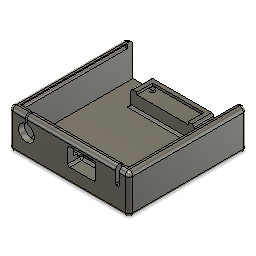
SyncLedStripHousing (Autodesk Fusion 360 design; units mm, degrees)
Autodesk Fusion 360 part; units mm, degrees
sketch "lipo battery" plane through (0, 0, 0) normal (0, 1, 0) x (1, 0, 0)
  line L0 (0, 0) -> (51, 0)
  line L1 (51, 0) -> (51, 34)
  line L2 (51, 34) -> (0, 34)
  line L3 (0, 34) -> (0, 0)
  dimension "d1" = 51
  dimension "d2" = 34
  constraint horizontal L0
  constraint vertical L1
  constraint horizontal L2
  constraint vertical L3
  constraint coincident L0.start L3.end
  measures "d1" distance of L0.start L0.end
  measures "d2" distance of L0.start L2.end
  measures "d159" distance of L0.start
extrude "Extrude1" add sketch "lipo battery" along normal blind 5.5 makes body 1
sketch "Lolin board" plane through (0, 0, 0) normal (0, 1, 0) x (1, 0, 0)
  line L0 (10, -5) -> (36, -5)
  line L1 (36, -5) -> (36, 45)
  line L2 (36, 45) -> (10, 45)
  line L3 (10, 45) -> (10, -5)
  line L4 (33.0596, -5) -> (25.0596, -5)
  line L5 (25.0596, -5) -> (25.0596, 1)
  line L6 (25.0596, 1) -> (33.0596, 1)
  line L7 (33.0596, 1) -> (33.0596, -5)
  line L8 (10, -5) -> (19.5, -5)
  line L9 (19.5, -5) -> (19.5, 3)
  line L10 (19.5, 3) -> (10, 3)
  line L11 (10, 3) -> (10, -5)
  circle A0 centre (12.4, 42.6) radius 1
  circle A1 centre (33.6, 3.5) radius 1
  dimension "d5" = 26
  dimension "d6" = 50
  dimension "d7" = 8
  dimension "d8" = 6
  dimension "d9" = 9.5
  dimension "d10" = 8
  dimension "d11" = 2
  dimension "d12" = 2
  constraint horizontal L0
  constraint vertical L1
  constraint horizontal L2
  constraint vertical L3
  constraint horizontal L4
  constraint vertical L5
  constraint horizontal L6
  constraint vertical L7
  constraint coincident L0 L4.start
  constraint horizontal L8
  constraint vertical L9
  constraint horizontal L10
  constraint vertical L11
  measures "d5" distance of L0.start L0.end
  measures "d6" distance of L0.start L2.end
  measures "d7" distance of L4.start L4.end
  measures "d8" distance of L4.start L6.end
  measures "d9" distance of L0.start L8.end
  measures "d10" distance of L0.start L10.end
  measures "d11" diameter of A0
  measures "d12" diameter of A1
extrude "Extrude2" add sketch "Lolin board" against normal blind 1.2 separate body makes body 2
extrude "Extrude3" add sketch "Lolin board" along normal blind 5.7 separate body contours L0 L3 L8 L9 L10 L11 makes body 3
extrude "Extrude4" add sketch "Lolin board" along normal blind 2.3 separate body contours L0 L4 L5 L6 L7 makes body 4
combine "Combine1" operation add target body 2 tool bodies 3 4
move_body "Move1" bodies 2 to x (1, 0, 0) y (0, 1, 0) z (0, 0, 1) at (0, 8, -3)
move_body "Move15" bodies 2 to x (1, 0, 0) y (0, 1, 0) z (0, 0, 1) at (3, 0, 6)
sketch "Housing" plane through (0, 0, 0) normal (0, 1, 0) x (1, 0, 0) in component "Housing"
  line L0 (-2, -10) -> (53, -10)
  line L1 (53, -10) -> (53, 44)
  line L2 (53, 44) -> (-2, 44)
  line L3 (-2, 44) -> (-2, -10)
  line L4 (10, 34) -> (42, 34)
  line L5 (42, 34) -> (42, 44)
  line L6 (42, 44) -> (10, 44)
  line L7 (10, 44) -> (10, 34)
  line L8 (10, -10) -> (42, -10)
  line L9 (42, -10) -> (42, -1)
  line L10 (42, -1) -> (10, -1)
  line L11 (10, -1) -> (10, -10)
  line L12 (-5, -13) -> (56, -13)
  line L13 (56, -13) -> (56, 47)
  line L14 (56, 47) -> (-5, 47)
  line L15 (-5, 47) -> (-5, -13)
  line L16 (39, -10) -> (25, -10)
  line L17 (25, -10) -> (25, -13)
  line L18 (25, -13) -> (39, -13)
  line L19 (39, -13) -> (39, -10)
  dimension "d121" = 3
  dimension "d122" = 14
  constraint horizontal L0
  constraint vertical L1
  constraint horizontal L2
  constraint vertical L3
  constraint horizontal L4
  constraint vertical L5
  constraint horizontal L6
  constraint vertical L7
  constraint coincident L2 L5.end
  constraint horizontal L8
  constraint vertical L9
  constraint horizontal L10
  constraint vertical L11
  constraint coincident L0 L8.start
  constraint horizontal L16
  constraint vertical L17
  constraint horizontal L18
  constraint vertical L19
  constraint coincident L0 L16.start
  measures "d122" distance of L16.start L16.end
extrude "Extrude1'" add sketch "Housing" against normal blind 3 separate body makes body 5 in component "Housing"
extrude "Extrude2'" add sketch "Housing" along normal blind 17 contours L0 L1 L2 L3 L6 L8 L12 L13 L14 L15 L17 L19 | L0 L8 L12 L16 L17 L18 L19 bodies 5 in component "Housing"
extrude "Extrude3'" add sketch "Housing" along normal blind 8 contours L0 L8 L9 L10 L11 L16 | L2 L4 L5 L6 L7 bodies 5 in component "Housing"
combine "Combine1'" operation cut target body 5 tool bodies 2 keep tools in component "Housing"
extrude "Extrude4'" add sketch "Housing" along normal blind 9 separate body contours L0 L8 L12 L16 L17 L18 L19 makes body 6 in component "Housing"
move_face "OffsetFaces1" offset 4 1 faces at (29.6667, 6, 10) on bodies 6 in component "Housing"
move_body "Move1'" bodies 6 to x (1, 0, 0) y (0, 1, 0) z (0, 0, 1) at (0, 5, 0) in component "Housing"
combine "Combine2" operation cut target body 5 tool bodies 6 in component "Housing"
sketch "Lid" plane through (0, 17, 0) normal (0, 1, 0) x (-1, 0, 0) in component "Lid"
  line L0 (-53, 10) -> (2, 10)
  line L1 (2, 10) -> (2, -44)
  line L2 (2, -44) -> (-53, -44)
  line L3 (-53, -44) -> (-53, 10)
  line L4 (5, 13) -> (-56, 13)
  line L5 (-56, 13) -> (-56, -47)
  line L6 (-56, -47) -> (5, -47)
  line L7 (5, -47) -> (5, 13)
  line L8 (5, -47) -> (-56, -47)
  line L9 (-56, -47) -> (-56, 13)
  line L10 (-56, 13) -> (5, 13)
  line L11 (5, 13) -> (5, -47)
  line L12 (2, -44) -> (-53, -44)
  line L13 (-53, -44) -> (-53, 10)
  line L14 (-53, 10) -> (2, 10)
  line L15 (2, 10) -> (2, -44)
  line L16 (-53, -44) -> (-53, -47)
  line L17 (2, -44) -> (2, -47)
  line L18 (-10, -44) -> (-42, -44)
  line L19 (-42, -44) -> (-42, -38)
  line L20 (-42, -38) -> (-10, -38)
  line L21 (-10, -38) -> (-10, -44)
  dimension "d132" = 3
  constraint horizontal L8
  constraint vertical L9
  constraint horizontal L10
  constraint vertical L11
  constraint coincident L4.end L5.start
  constraint coincident L6.end L7.start
  constraint coincident L2.end L3.start
  constraint coincident L6 L16.end
  constraint perpendicular L6 L16
  constraint coincident L1.end L2.start
  constraint coincident L6 L17.end
  constraint perpendicular L6 L17
  constraint horizontal L18
  constraint vertical L19
  constraint horizontal L20
  constraint vertical L21
  constraint coincident L2 L18.start
extrude "Extrude1''" add sketch "Lid" against normal blind 3 separate body contours L0 L1 L2 L3 L12 L13 L14 L15 L19 L20 L21 | L2 L12 L18 L19 L20 L21 makes body 7 in component "Lid"
extrude "Extrude2''" add sketch "Lid" against normal blind 17 contours L2 L6 L8 L12 L16 L17 L18 bodies 7 in component "Lid"
sketch "Sketch2" plane through (0, 0, 10) normal (0, 0, 1) x (1, 0, 0) in component "Lid"
  line L0 (53, 17) -> (-2, 17)
  line L1 (-2, 17) -> (-2, 14)
  line L2 (-2, 14) -> (53, 14)
  line L3 (53, 14) -> (53, 17)
  circle A0 centre (-2, 15.5) radius 1
  circle A1 centre (53, 15.5) radius 1
  dimension "d137" = 2
  dimension "d138" = 2
  constraint midpoint L1 A0.centre
  constraint midpoint L3 A1.centre
  measures "d137" diameter of A0
  measures "d138" diameter of A1
extrude "Extrude3''" add sketch "Sketch2" against normal blind 54 contours L3 A1 | L3 A1 | L1 A0 | L1 A0 bodies 7 in component "Lid"
combine "Combine3" operation cut target body 5 tool bodies 7 keep tools in component "Housing"
move_face "OffsetFaces1'" offset -0.5 1 faces at (-2, 10.3333, -46) on bodies 7 in component "Lid"
move_face "MoveFace1" to x (1, 0, 0) y (0, 1, 0) z (0, 0, 1) at (0.5, 0, 0) 1 faces at (-2.9749, 15.2775, -8) on bodies 7 in component "Lid"
move_face "OffsetFaces2" offset -0.5 1 faces at (53, 10.3333, -46) on bodies 7 in component "Lid"
move_face "MoveFace2" to x (1, 0, 0) y (0, 1, 0) z (0, 0, 1) at (-0.5, 0, 0) 1 faces at (53.4562, 14.6101, -26) on bodies 7 in component "Lid"
move_face "OffsetFaces3" offset -0.5 1 faces at (34.5, 15.1667, 10) on bodies 7 in component "Lid"
fillet "Fillet1" radius 2 4 edges at (-5, 7, -47) (-5, 7, 13) (56, 7, 13) (56, 7, -47) on bodies 5 in component "Housing"
fillet "Fillet2" radius 2 8 edges at (55.4142, -3, 12.4142) (25.5, -3, 13) (-4.4142, -3, 12.4142) (-5, -3, -17) (-4.4142, -3, -46.4142) (25.5, -3, -47) (55.4142, -3, -46.4142) (56, -3, -17) on bodies 5 in component "Housing"
fillet "Fillet1'" radius 1 4 edges at (53.5, 15.5, -44) (-2.5, 15.5, -44) (-2.5, 15.5, 9.5) (53.5, 15.5, 9.5) on bodies 7 in component "Lid"
fillet "Fillet3" radius 1 4 edges at (39, 5, 9.5) (39, 14, 11.5) (25, 14, 11.5) (25, 5, 9.5) on bodies 5 in component "Housing"
fillet "Fillet4" radius 1 4 edges at (42, 8, -39) (42, 8, 5.5) (10, 8, 5.5) (10, 8, -39) on bodies 5 in component "Housing"
fillet "Fillet5" radius 1 6 edges at (42, 0, -39) (26, 0, -34) (42, 0, 5.5) (26, 0, 1) (10, 0, 5.5) (10, 0, -39) on bodies 5 in component "Housing"
fillet "Fillet6" radius 1 5 edges at (39, 6.4, 6) (38.7071, 5.2929, 6) (32, 5, 6) (25.2929, 5.2929, 6) (25, 6.4, 6) on bodies 5 in component "Housing"
extrude "Extrude4''" add sketch "Lid" against normal blind 8.5 contours L2 L12 L18 L19 L20 L21 bodies 7 in component "Lid"
draft "Draft1" angle 5 neutral plane through (42, 17, -44) pull (0, 0, 1) 1 faces at (31.3333, 8.5, -42) on bodies 7 in component "Lid"
fillet "Fillet2'" radius 1 5 edges at (10, 8.7625, -41) (26, 9.0249, -38) (42, 8.7625, -41) (42, 11.5125, -38) (10, 11.5125, -38) on bodies 7 in component "Lid"
fillet "Fillet3'" radius 1 7 edges at (10, 14, -41.5) (10.2929, 14, -38.2929) (26, 14, -38) (41.7071, 14, -38.2929) (42, 14, -41.5) (47.25, 14, -44) (4.25, 14, -44) on bodies 7 in component "Lid"
fillet "Fillet4'" radius 2 1 edges at (25.5, 17, -47) on bodies 7 in component "Lid"
fillet "Fillet7" radius 2 9 edges at (-2.5, 17, -47) (-4.4142, 17, -46.4142) (-5, 17, -17) (-4.4142, 17, 12.4142) (25.5, 17, 13) (55.4142, 17, 12.4142) (56, 17, -17) (55.4142, 17, -46.4142) (53.5, 17, -47) on bodies 5 in component "Housing"
sketch "Sketch1" plane through (0, 17, 0) normal (0, 1, 0) x (-1, 0, 0) in component "Holder"
  line L0 (-52.5, -45) -> (1.5, -45)
  line L1 (1.5, -45) -> (1.5, 9.5)
  line L2 (1.5, 9.5) -> (-52.5, 9.5)
  line L3 (-52.5, 9.5) -> (-52.5, -45)
  line L4 (-56, -15) -> (5, -15)
  line L5 (5, -15) -> (5, 11.0228)
  line L6 (3, 13.0228) -> (-54, 13.0228)
  line L7 (-56, 11.0228) -> (-56, -15)
  arc A0 (5, 11.0228) -> (3, 13.0228) centre (3, 11.0228) ccw
  arc A1 (-54, 13.0228) -> (-56, 11.0228) centre (-54, 11.0228) ccw
  line L8 (7, -15) -> (7, 11.0228)
  arc A2 (7, 11.0228) -> (3, 15.0228) centre (3, 11.0228) ccw
  line L9 (3, 15.0228) -> (-54, 15.0228)
  arc A3 (-54, 15.0228) -> (-58, 11.0228) centre (-54, 11.0228) ccw
  line L10 (-58, 11.0228) -> (-58, -15)
  line L11 (7, -15) -> (-58, -15)
  circle A4 centre (-10, -5) radius 1.5
  circle A5 centre (-41, -5) radius 1.5
  line L12 (3, -15) -> (3, 9.0228)
  line L13 (1, 11.0228) -> (-52, 11.0228)
  line L14 (-54, 9.0228) -> (-54, -15)
  arc A6 (3, 9.0228) -> (1, 11.0228) centre (1, 9.0228) ccw
  arc A7 (-52, 11.0228) -> (-54, 9.0228) centre (-52, 9.0228) ccw
  dimension "d159" = 61
  dimension "d160" = 2
  dimension "d161" = 2
  dimension "d162" = 2
  dimension "d163" = 3
  dimension "d164" = 3
  dimension "d172" = 2
  dimension "d173" = 2
  constraint horizontal L4
  constraint vertical L5
  constraint horizontal L6
  constraint vertical L7
  constraint tangent L5 A0
  constraint tangent L6 A0
  constraint tangent L6 A1
  constraint tangent L7 A1
  constraint perpendicular L10 L11
  constraint parallel L5 L12
  constraint parallel L6 L13
  constraint parallel L7 L14
  constraint tangent L12 A6
  constraint tangent L13 A6
  constraint tangent L13 A7
  constraint tangent L14 A7
  measures "d159" distance of L4.start L4.end
  measures "d160" radius of A0
  measures "d161" radius of A1
  measures "d163" diameter of A4
  measures "d164" diameter of A5
  measures "d172" radius of A6
  measures "d173" radius of A7
extrude "Extrude3'''" add sketch "Sketch1" along normal blind 2 separate body contours L4 L5 L6 L7 A0 A1 L11 L12 L13 L14 A6 A7 | L5 L6 L7 A0 A1 L8 A2 L9 A3 L10 L11 makes body 8 in component "Holder"
extrude "Extrude2'''" add sketch "Sketch1" against normal blind 20 separate body contours L5 L6 L7 A0 A1 L8 A2 L9 A3 L10 L11 makes body 9 in component "Holder"
extrude "Extrude1'''" add sketch "Sketch1" along normal blind 3 separate body contours L1 L2 L3 L4 L11 L12 L13 L14 A6 A7 | L1 L2 L3 L4 L11 | L4 L5 L6 L7 A0 A1 L11 L12 L13 L14 A6 A7 | L5 L6 L7 A0 A1 L8 A2 L9 A3 L10 L11 makes body 10 in component "Holder"
move_body "Move1''" bodies 8 to x (1, 0, 0) y (0, 1, 0) z (0, 0, 1) at (0, -22, 0) in component "Holder"
combine "Combine1''" operation add target body 8 tool bodies 9 10 in component "Holder"
combine "Combine2'" operation cut target body 8 tool bodies 5 7 keep tools in component "Holder"
move_face "OffsetFaces1''" offset -0.5 3 faces at (56, 3.6667, 2.3485) (-5, 3.6667, -6.3257) (16, 10.3333, 13.0228) on bodies 8 in component "Holder"
move_face "OffsetFaces2'" offset -0.5 1 faces at (16.6667, -3, 12.6894) on bodies 8 in component "Holder"
fillet "Fillet1''" radius 2 5 edges at (-7, -5, -1.9886) (-5.8284, -5, 13.8512) (25.5, -5, 15.0228) (56.8284, -5, 13.8512) (58, -5, -1.9886) on bodies 8 in component "Holder"
fillet "Fillet2''" radius 2 5 edges at (-7, 20, -1.9886) (-5.8284, 20, 13.8512) (25.5, 20, 15.0228) (56.8284, 20, 13.8512) (58, 20, -1.9886) on bodies 8 in component "Holder"
fillet "Fillet3''" radius 2 5 edges at (-5.5, -3.5, -1.7386) (-4.9142, -3.5, 12.937) (25.5, -3.5, 13.5228) (55.9142, -3.5, 12.937) (56.5, -3.5, -1.7386) on bodies 8 in component "Holder"
fillet "Fillet4''" radius 2 5 edges at (-5.5, 17, -1.7386) (-4.9142, 17, 12.937) (25.5, 17, 13.5228) (55.9142, 17, 12.937) (56.5, 17, -1.7386) on bodies 8 in component "Holder"
fillet "Fillet5'" radius 1 5 edges at (-3, -5, -2.9886) (-2.4142, -5, 10.437) (25.5, -5, 11.0228) (53.4142, -5, 10.437) (54, -5, -2.9886) on bodies 8 in component "Holder"
chamfer "Chamfer1" distance 2 angle 45 1 edges at (11.3985, 17, -4.4576) on bodies 8 in component "Holder"
chamfer "Chamfer2" distance 2 angle 45 1 edges at (42.3985, 17, -4.4576) on bodies 8 in component "Holder"
fillet "Fillet7'" radius 1 13 edges at (54, -3.75, -15) (54.2929, -4.7071, -15) (55.5, -5, -15) (57.4142, -4.4142, -15) (58, 7.5, -15) (57.4142, 19.4142, -15) (25.5, 20, -15) (-6.4142, 19.4142, -15) (-7, 7.5, -15) (-6.4142, -4.4142, -15) (-4.5, -5, -15) (-3.2929, -4.7071, -15) (-3, -3.75, -15) on bodies 8 in component "Holder"
fillet "Fillet8" radius 0.6 16 edges at (56.5, 6.75, -15) (56.0811, -2.7247, -15) (54.7462, -3.4846, -14.967) (54.134, -3.5, -14.5) (54, -3.5, -2.4886) (53.4142, -3.5, 10.437) (25.5, -3.5, 11.0228) (-2.4142, -3.5, 10.437) (-3, -3.5, -2.4886) (-3.134, -3.5, -14.5) (-3.7462, -3.4846, -14.967) (-5.0811, -2.7247, -15) (-5.5, 6.75, -15) (-4.9142, 16.4142, -15) (25.5, 17, -15) (55.9142, 16.4142, -15) on bodies 8 in component "Holder"
sketch "Buttonhole" plane through (0, 0, 10) normal (0, 0, -1) x (-1, 0, 0)
  arc A0 (-43, 0) -> (-42, 1) centre (-43, 1) ccw
  line L0 (-42, 1) -> (-42, 7)
  arc A1 (-41, 8) -> (-42, 7) centre (-41, 7) ccw
  line L1 (-41, 8) -> (-39, 8)
  line L2 (-39, 8) -> (-39, 13)
  arc A2 (-38, 14) -> (-39, 13) centre (-38, 13) ccw
  line L3 (-38, 14) -> (-26, 14)
  arc A3 (-25, 13) -> (-26, 14) centre (-26, 13) ccw
  line L4 (-25, 13) -> (-25, 8)
  line L5 (-25, 8) -> (-11, 8)
  arc A4 (-10, 7) -> (-11, 8) centre (-11, 7) ccw
  line L6 (-10, 7) -> (-10, 1)
  arc A5 (-10, 1) -> (-9, 0) centre (-9, 1) ccw
  line L7 (-9, 0) -> (2, 0)
  line L8 (2, 0) -> (2, 14.5)
  arc A6 (2, 14.5) -> (2, 16.5) centre (2, 15.5) ccw
  line L9 (2, 17) -> (-53, 17)
  line L10 (-53, 17) -> (-53, 16.5)
  arc A7 (-53, 16.5) -> (-53, 14.5) centre (-53, 15.5) ccw
  line L11 (-53, 14.5) -> (-53, 0)
  line L12 (-53, 0) -> (-43, 0)
  line L13 (1.0045, 14.0126) -> (-8.9955, 14.0126)
  line L14 (-8.9955, 14.0126) -> (-8.9955, 4.0126)
  line L15 (-8.9955, 4.0126) -> (1.0045, 4.0126)
  line L16 (1.0045, 4.0126) -> (1.0045, 14.0126)
  circle A8 centre (-3.9955, 9.0126) radius 4
  line L17 (2, 16.5) -> (2, 17)
  line L18 (-51.0774, 17) -> (-49.0774, 17)
  line L19 (-49.0774, 17) -> (-49.0774, 9.5)
  line L20 (-49.5774, 9) -> (-50.5774, 9)
  line L21 (-51.0774, 9.5) -> (-51.0774, 17)
  arc A9 (-51.0774, 9.5) -> (-50.5774, 9) centre (-50.5774, 9.5) ccw
  arc A10 (-49.5774, 9) -> (-49.0774, 9.5) centre (-49.5774, 9.5) ccw
  line L22 (-4.4955, 12.506) -> (-3.4955, 12.506)
  line L23 (-3.4955, 12.506) -> (-3.4955, 17.506)
  line L24 (-3.4955, 17.506) -> (-4.4955, 17.506)
  line L25 (-4.4955, 17.506) -> (-4.4955, 12.506)
  line L26 (-4.4955, 12.506) -> (-3.4955, 17.506) construction
  line L27 (-3.4955, 12.506) -> (-4.4955, 17.506) construction
  point P0 (-51.0774, 9)
  point P1 (-3.9955, 15.006)
  dimension "d204" = 10
  dimension "d205" = 10
  dimension "d206" = 8
  dimension "d209" = 2
  dimension "d210" = 8
  dimension "d211" = 0.5
  dimension "d212" = 0.5
  dimension "d215" = 1
  dimension "d216" = 5
  constraint horizontal L13
  constraint vertical L14
  constraint horizontal L15
  constraint vertical L16
  constraint horizontal L18
  constraint vertical L19
  constraint horizontal L20
  constraint vertical L21
  constraint coincident L9 L18.start
  constraint coincident P0 L20
  constraint coincident P0 L21
  constraint tangent L20 A9
  constraint tangent L21 A9
  constraint tangent L19 A10
  constraint tangent L20 A10
  constraint horizontal L22
  constraint perpendicular L22 L23
  constraint parallel L22 L24
  constraint parallel L23 L25
  constraint coincident L26 P1
  constraint coincident L27 P1
  measures "d204" distance of L13.start L13.end
  measures "d205" distance of L13.start L15.end
  measures "d206" diameter of A8
  measures "d209" distance of L18.start L18.end
  measures "d210" distance of L18.start P0
  measures "d211" radius of A9
  measures "d212" radius of A10
  measures "d215" distance of L23.end L24.end
  measures "d216" distance of L22.end L23.end
extrude "Extrude5" cut sketch "Buttonhole" along normal mid plane 8 contours A8 L22 L23 L25 | A8 L22 L23 L25 bodies 5 in component "Housing"
extrude "Extrude6" cut sketch "Buttonhole" along normal mid plane 8 contours L9 L18 L19 L20 L21 A9 A10 bodies 5 in component "Housing"
extrude "Extrude7" cut sketch "Buttonhole" along normal mid plane 6 contours L9 L23 L24 L25 | L9 L13 L23 L25 | L13 A8 L23 L25 | A8 L22 L23 L25 picked at (-4.0512, 12.6737) bodies 5 in component "Housing"
component "Housing" placed x (1, 0, 0) y (0, 1, 0) z (0, 0, 1) at (0, 0, 0)
component "Lid" placed x (1, 0, 0) y (0, 1, 0) z (0, 0, 1) at (0, 0, 0)
component "Holder" placed x (1, 0, 0) y (0, 1, 0) z (0, 0, 1) at (0, 0, 0)
named bodies: "lipo battery", "Lolin board", "Housing", "Lid", "Holder"
